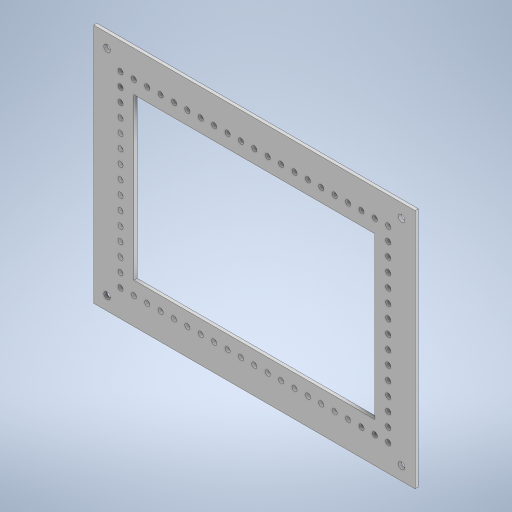
# Autodesk Inventor part: Middle plate
Saved by Autodesk Inventor 2023.4 (Build 274418000, 418)
## iProperties
Created: 2023-12-24
Part Number: Middle plate
Material: Generic
Document SubType Name: Sheet Metal
Designer: amrom
Density: 1 g/cm^3
Sheet Metal Rule: Default
Appearance: Default
Author: amrom
Autodesk Inventor part; units mm, degrees
ref_plane "YZ Plane" through (0, 0, 0) normal (1, 0, 0) x (0, 1, 0)
ref_plane "XZ Plane" through (0, 0, 0) normal (0, 1, 0) x (-1, 0, 0)
ref_plane "XY Plane" through (0, 0, 0) normal (0, 0, 1) x (1, 0, 0)
sketch "Sketch1" plane through (0, 0, 0) normal (0, 0, 1) x (1, 0, 0)
  line L0 (0, 0) -> (228.6, 0)
  line L1 (228.6, 0) -> (228.6, 152.4)
  line L2 (228.6, 152.4) -> (0, 152.4)
  line L3 (0, 152.4) -> (0, 0)
  line L4 (-38.1, -38.1) -> (266.7, -38.1)
  line L5 (266.7, -38.1) -> (266.7, 190.5)
  line L6 (266.7, 190.5) -> (-38.1, 190.5)
  line L7 (-38.1, 190.5) -> (-38.1, -38.1)
  dimension "d0" = 228.6
  dimension "d1" = 152.4
  dimension "d2" = 38.1
  measures "d0" distance of L2.end L1.end
  measures "d1" distance of L1.end L0.end
  measures "d2" distance between parallel lines of L3 L7
extrude "Plate1" add sketch "Sketch1" along normal blind 3.048
sketch "Sketch2" plane through (0, 0, 3.048) normal (0, 0, 1) x (1, 0, 0)
  circle A0 centre (-12.7, -12.7) radius 2.5019
  line L0 (-38.1, -38.1) -> (-38.1, 190.5) projected
  line L1 (228.6, 0) -> (0, 0) projected
  line L2 (0, 0) -> (0, 152.4) projected
  circle A1 centre (0, -12.7) radius 2.5019
  circle A2 centre (12.7, -12.7) radius 2.5019
  circle A3 centre (25.4, -12.7) radius 2.5019
  circle A4 centre (38.1, -12.7) radius 2.5019
  circle A5 centre (50.8, -12.7) radius 2.5019
  circle A6 centre (63.5, -12.7) radius 2.5019
  circle A7 centre (76.2, -12.7) radius 2.5019
  circle A8 centre (88.9, -12.7) radius 2.5019
  circle A9 centre (101.6, -12.7) radius 2.5019
  circle A10 centre (114.3, -12.7) radius 2.5019
  circle A11 centre (127, -12.7) radius 2.5019
  circle A12 centre (139.7, -12.7) radius 2.5019
  circle A13 centre (152.4, -12.7) radius 2.5019
  circle A14 centre (165.1, -12.7) radius 2.5019
  circle A15 centre (177.8, -12.7) radius 2.5019
  circle A16 centre (190.5, -12.7) radius 2.5019
  circle A17 centre (203.2, -12.7) radius 2.5019
  circle A18 centre (215.9, -12.7) radius 2.5019
  circle A19 centre (241.3, -12.7) radius 2.5019
  circle A20 centre (241.3, 0) radius 2.5019
  circle A21 centre (241.3, 12.7) radius 2.5019
  circle A22 centre (241.3, 25.4) radius 2.5019
  circle A23 centre (241.3, 38.1) radius 2.5019
  circle A24 centre (241.3, 50.8) radius 2.5019
  circle A25 centre (241.3, 63.5) radius 2.5019
  circle A26 centre (241.3, 76.2) radius 2.5019
  circle A27 centre (241.3, 88.9) radius 2.5019
  circle A28 centre (241.3, 101.6) radius 2.5019
  circle A29 centre (241.3, 114.3) radius 2.5019
  circle A30 centre (241.3, 127) radius 2.5019
  circle A31 centre (241.3, 165.1) radius 2.5019
  line L3 (0, 152.4) -> (228.6, 152.4) projected
  circle A32 centre (241.3, 139.7) radius 2.5019
  circle A33 centre (228.6, 165.1) radius 2.5019
  circle A34 centre (215.9, 165.1) radius 2.5019
  circle A35 centre (203.2, 165.1) radius 2.5019
  circle A36 centre (190.5, 165.1) radius 2.5019
  circle A37 centre (177.8, 165.1) radius 2.5019
  circle A38 centre (165.1, 165.1) radius 2.5019
  circle A39 centre (152.4, 165.1) radius 2.5019
  circle A40 centre (139.7, 165.1) radius 2.5019
  circle A41 centre (127, 165.1) radius 2.5019
  circle A42 centre (114.3, 165.1) radius 2.5019
  circle A43 centre (101.6, 165.1) radius 2.5019
  circle A44 centre (88.9, 165.1) radius 2.5019
  circle A45 centre (76.2, 165.1) radius 2.5019
  circle A46 centre (63.5, 165.1) radius 2.5019
  circle A47 centre (50.8, 165.1) radius 2.5019
  circle A48 centre (38.1, 165.1) radius 2.5019
  circle A49 centre (25.4, 165.1) radius 2.5019
  circle A50 centre (12.7, 165.1) radius 2.5019
  circle A51 centre (-12.7, 165.1) radius 2.5019
  circle A52 centre (-12.7, 152.4) radius 2.5019
  circle A53 centre (-12.7, 139.7) radius 2.5019
  circle A54 centre (-12.7, 127) radius 2.5019
  circle A55 centre (-12.7, 114.3) radius 2.5019
  circle A56 centre (-12.7, 101.6) radius 2.5019
  circle A57 centre (-12.7, 88.9) radius 2.5019
  circle A58 centre (-12.7, 76.2) radius 2.5019
  circle A59 centre (-12.7, 63.5) radius 2.5019
  circle A60 centre (-12.7, 50.8) radius 2.5019
  circle A61 centre (-12.7, 38.1) radius 2.5019
  circle A62 centre (-12.7, 25.4) radius 2.5019
  circle A63 centre (-12.7, 12.7) radius 2.5019
  circle A64 centre (-12.7, 0) radius 2.5019
  circle A65 centre (0, 165.1) radius 2.5019
  circle A66 centre (241.3, 152.4) radius 2.5019
  circle A67 centre (228.6, -12.7) radius 2.5019
  dimension "d4" = 5.0038
  dimension "d6" = 12.7
  dimension "d7" = 12.7
  dimension "d10" = 12.7
  dimension "d17" = 5.0038
  dimension "d18" = 25.4
  dimension "d19" = 12.7
  dimension "d22" = 12.7
  dimension "d27" = 5.0038
  dimension "d30" = 25.4
  dimension "d31" = 12.7
  dimension "d34" = 12.7
  dimension "d39" = 5.0038
  dimension "d40" = 25.4
  dimension "d41" = 12.7
  dimension "d44" = 12.7
  constraints: 68 centre point, 2 horizontal, 2 vertical, 128 other
  measures "d4" diameter of A0
  measures "d6" distance from line of L1 A0.centre
  measures "d7" distance from line of A0.centre L2
  measures "d10" distance of A0.centre A1.centre
  measures "d17" diameter of A19
  measures "d18" distance of A18.centre A19.centre
  measures "d19" distance from line of L1 A19.centre
  measures "d22" distance of A19.centre A20.centre
  measures "d27" diameter of A31
  measures "d30" distance of A32.centre A31.centre
  measures "d31" distance from line of L3 A31.centre
  measures "d34" distance of A31.centre A33.centre
  measures "d39" diameter of A51
  measures "d40" distance of A50.centre A51.centre
  measures "d41" distance from line of L3 A51.centre
  measures "d44" distance of A51.centre A52.centre
extrude "Extrusion1" cut sketch "Sketch2" against normal blind 25.4
sketch "Sketch3" plane through (0, 0, 3.048) normal (0, 0, 1) x (1, 0, 0)
  circle A0 centre (-25.4, -25.4) radius 3.175
  line L0 (-38.1, -38.1) -> (-38.1, 190.5) projected
  line L1 (266.7, -38.1) -> (-38.1, -38.1) projected
  circle A1 centre (-25.4, 177.8) radius 3.175
  line L2 (-38.1, 190.5) -> (266.7, 190.5) projected
  circle A2 centre (254, 177.8) radius 3.175
  line L3 (266.7, 190.5) -> (266.7, -38.1) projected
  circle A3 centre (254, -25.4) radius 3.175
  point P0 (0, 0)
  dimension "d49" = 6.35
  dimension "d50" = 12.7
  dimension "d51" = 12.7
  dimension "d52" = 6.35
  dimension "d53" = 12.7
  dimension "d54" = 12.7
  dimension "d55" = 6.35
  dimension "d56" = 12.7
  dimension "d57" = 12.7
  dimension "d58" = 6.35
  dimension "d59" = 12.7
  dimension "d60" = 12.7
  constraints: 4 centre point
  measures "d49" diameter of A0
  measures "d50" distance from line of L0 A0.centre
  measures "d51" distance from line of L1 A0.centre
  measures "d52" diameter of A1
  measures "d53" distance from line of L2 A1.centre
  measures "d54" distance from line of L0 A1.centre
  measures "d55" diameter of A2
  measures "d56" distance from line of L2 A2.centre
  measures "d57" distance from line of L3 A2.centre
  measures "d58" diameter of A3
  measures "d59" distance from line of L3 A3.centre
  measures "d60" distance from line of L1 A3.centre
extrude "Extrusion2" cut sketch "Sketch3" against normal blind 25.4 contours A0 | A1 | A2 | A3
equation "\"d3\" = Thickness"
equation "\"BendRadius\" = Thickness"
equation "\"BendReliefWidth\" = Thickness"
equation "\"BendReliefDepth\" = 0.5 * Thickness"
equation "\"CornerReliefSize\" = 4 * Thickness"
equation "\"MinimumRemnant\" = 2 * Thickness"
equation "\"TransitionRadius\" = BendRadius"
equation "\"JacobiRadiusSize\" = BendRadius"
equation "\"GapSize\" = Thickness"
equation "\"Thickness\" = 3.048"
body "Solid1"
